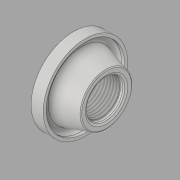
# Autodesk Inventor part: AN871-8D
Saved by Autodesk Inventor 2019 (Build 230136000, 136)
## iProperties
Created: 2018-12-01
Part Number: AN871-8D
Material: Aluminum 2014-T6
Document SubType Name: Modeling
Designer: erics
Density: 2.78927 g/cm^3
Appearance: Satin
Mass: 32.7822 g
Surface Area: 57.3289 cm^2
Volume: 11.753 cm^3
Author: erics
Autodesk Inventor part; units mm, degrees
ref_plane "YZ Plane" through (0, 0, 0) normal (1, 0, 0) x (0, 1, 0)
ref_plane "XZ Plane" through (0, 0, 0) normal (0, 1, 0) x (-1, 0, 0)
ref_plane "XY Plane" through (0, 0, 0) normal (0, 0, 1) x (1, 0, 0)
sketch "Sketch1" plane through (0, 0, 0) normal (0, 0, 1) x (1, 0, 0)
  line L0 (0, 22.225) -> (0, 9.525)
  line L1 (0, 9.525) -> (14.8209, 9.525)
  line L2 (15.0622, 9.7663) -> (16.2326, 9.7663)
  line L3 (16.8925, 10.1473) -> (17.4498, 11.1125)
  line L4 (17.4498, 11.1125) -> (17.4498, 13.0905)
  line L5 (17.0705, 13.6041) -> (4.2959, 17.5326)
  arc A0 (4.7625, 20.6375) -> (4.2959, 17.5326) centre (4.7625, 19.05) ccw
  line L6 (4.7625, 20.6375) -> (6.35, 20.6375)
  line L7 (6.35, 20.6375) -> (6.35, 22.225)
  line L8 (6.35, 22.225) -> (0, 22.225)
  arc A1 (16.2326, 9.7663) -> (16.8925, 10.1473) centre (16.2326, 10.5283) ccw
  line L9 (14.8209, 9.525) -> (15.0622, 9.7663)
  line L10 (-5.715, 0) -> (34.29, 0) projected
  line L11 (17.0705, 13.6041) -> (17.4498, 13.0905)
  point P0 (0, 0)
  point P1 (17.4498, 13.4874)
  dimension "d0" = 22.225
  dimension "d1" = 17.4498
  dimension "d2" = 13.4874
  dimension "d3" = 1.5875
  dimension "d4" = 1.5875
  dimension "d5" = 6.35
  dimension "d6" = 3.175
  dimension "d7" = 9.525
  dimension "d8" = 60
  dimension "d9" = 11.1125
  dimension "d10" = 9.7663
  dimension "d12" = 0.762
  dimension "d13" = 45
  dimension "d14" = 2.3876
  dimension "d18" = 0.3969
  dimension "d19" = 0.3969
  constraints: 22 end point, 4 point on circle, 4 tangent, 2 centre point, 2 horizontal, 2 parallel, 2 perpendicular, 2 point on line, 1 vertical, 1 vertical alignment
  measures "d0" distance from line of L8 point (0, 0)
  measures "d1" distance between parallel lines of L4 L0
  measures "d2" vertical distance of point (0, 0) point (17.45, 13.487)
  measures "d3" distance of L6.end L7.end
  measures "d4" radius of A0
  measures "d5" distance of L7.end L0.start
  measures "d6" distance edge to line of A0 L0
  measures "d7" distance from line of point (0, 0) L1
  measures "d8" angle of L2 L3
  measures "d9" vertical distance of point (0, 0) L3.end
  measures "d10" distance from line of point (0, 0) L2
  measures "d12" radius of A1
  measures "d13" angle of L2 L9
  measures "d14" distance from line of L4 L2.start
  measures "d18" distance of L5.start point (17.45, 13.487)
  measures "d19" distance of L4.end point (17.45, 13.487)
revolve "Revolution1" add sketch "Sketch1" angle 360 about axis through (-10, 0, 0) along (1, 0, 0)
thread "Thread1" size "3/4-16 UNF" class "2B" standard "ANSI Unified Screw Threads" full length
equation "\"d0\" = 0.5 * AN871_A"
equation "\"d1\" = AN871_C"
equation "\"d2\" = 0.5 * AN871_B"
equation "\"d7\" = 0.5 * AN871_T"
equation "\"d9\" = 0.5 * AND10050_A"
equation "\"d10\" = 0.5 * AND10050_D"
equation "\"d14\" = AND10050_E"
equation "\"d19\" = d18"
equation "\"AN871_A\" = 44.45"
equation "\"AN871_B\" = 26.9748"
equation "\"AN871_C\" = 17.4498"
equation "\"AN871_T\" = 19.05"
equation "\"AND10050_A\" = 22.225"
equation "\"AND10050_D\" = 19.5326"
equation "\"AND10050_E\" = 2.3876"
body "Solid1"
